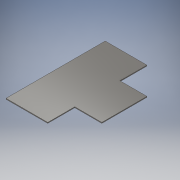
# Autodesk Inventor part: top_bottom_rev2
Saved by Autodesk Inventor 2017 (Build 210142000, 142)
## iProperties
Created: 2016-12-07
Part Number: top_bottom_rev2
Material: Steel, Mild
Document SubType Name: Sheet Metal
Designer: Robert.Chapman
Density: 7.85 g/cm^3
Sheet Metal Rule: Default
Appearance: Semi-Polished
Mass: 7233.5 g
Surface Area: 4003.22 cm^2
Volume: 921.465 cm^3
Author: Robert.Chapman
Autodesk Inventor part; units mm, degrees
ref_plane "YZ Plane" through (0, 0, 0) normal (1, 0, 0) x (0, 1, 0)
ref_plane "XZ Plane" through (0, 0, 0) normal (0, 1, 0) x (-1, 0, 0)
ref_plane "XY Plane" through (0, 0, 0) normal (0, 0, 1) x (1, 0, 0)
sketch "Sketch1" plane through (0, 0, 0) normal (0, 1, 0) x (-1, 0, 0)
  line L0 (58.3565, 287.7551) -> (-176.5935, 287.7551)
  line L1 (-176.5935, -271.0449) -> (58.3565, -271.0449)
  line L2 (58.3565, -271.0449) -> (58.3565, 287.7551)
  line L3 (-176.5935, 287.7551) -> (-176.5935, 135.3551)
  line L4 (-176.5935, 135.3551) -> (-328.9935, 135.3551)
  line L5 (-328.9935, -118.6449) -> (-176.5935, -118.6449)
  line L6 (-176.5935, -118.6449) -> (-176.5935, -271.0449)
  line L7 (-328.9935, 135.3551) -> (-328.9935, 76.6176)
  line L8 (-328.9935, -59.9074) -> (-328.9935, -118.6449)
  line L9 (-328.9935, -59.9074) -> (-328.9935, 76.6176)
  dimension "d3" = 558.8
  dimension "d4" = 234.95
  dimension "d5" = 152.4
  dimension "d6" = 152.4
  dimension "d11" = 152.4
  dimension "d12" = 234.95
  measures "d3" distance of L1.end L0.start
  measures "d4" distance of L0.start L0.end
  measures "d5" distance of L3.end L4.end
  measures "d6" distance of L0.end L3.end
  measures "d11" distance of L5.end L1.start
  measures "d12" distance of L1.start L1.end
extrude "Plate1" add sketch "Sketch1" along normal blind 4.7625
equation "\"BendRadius\" = Thickness"
equation "\"BendReliefWidth\" = Thickness"
equation "\"BendReliefDepth\" = 0.5 * Thickness"
equation "\"CornerReliefSize\" = 4 * Thickness"
equation "\"MinimumRemnant\" = 2 * Thickness"
equation "\"TransitionRadius\" = BendRadius"
equation "\"JacobiRadiusSize\" = BendRadius"
equation "\"GapSize\" = Thickness"
equation "\"d9\" = BendRadius"
equation "\"Thickness\" = 4.7625"
body "Solid1"
